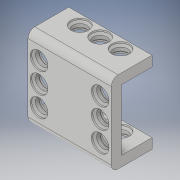
# Autodesk Inventor part: XL320_connecter
Saved by Autodesk Inventor 2018 (Build 220112000, 112)
## iProperties
Created: 2018-01-21
Part Number: XL320_connecter
Material: Generic
Document SubType Name: Modeling
Designer: wlpeng
Density: 1 g/cm^3
Appearance: Default
Author: wlpeng
Autodesk Inventor part; units mm, degrees
ref_plane "YZ Plane" through (0, 0, 0) normal (1, 0, 0) x (0, 1, 0)
ref_plane "XZ Plane" through (0, 0, 0) normal (0, 1, 0) x (-1, 0, 0)
ref_plane "XY Plane" through (0, 0, 0) normal (0, 0, 1) x (1, 0, 0)
sketch "Sketch2" plane through (0, 0, 0) normal (1, 0, 0) x (0, 1, 0)
  line L0 (3, -3) -> (3, -12)
  line L1 (3, -12) -> (0, -12)
  line L2 (0, -12) -> (0, 0)
  line L3 (21, -3) -> (3, -3)
  line L4 (0, -3) -> (0, 0)
  line L5 (21, -3) -> (21, -12)
  line L6 (21, -12) -> (24, -12)
  line L7 (24, -12) -> (24, 0)
  line L8 (24, 0) -> (0, 0)
  dimension "d2" = 24
  dimension "d3" = 3
  dimension "d4" = 12
  constraints: 18 end point, 3 parallel, 1 perpendicular
  measures "d2" distance of L2.end L7.end
  measures "d3" distance of L5.end L6.end
  measures "d4" distance of L1.end L2.end
extrude "Extrusion1" add sketch "Sketch2" along normal blind 24.5
sketch "Sketch3" plane through (0, 24, 0) normal (0, 1, 0) x (1, 0, 0)
  circle A0 centre (12.25, 9) radius 2.05
  line L0 (0, 12) -> (0, 0) projected
  line L1 (0, 0) -> (24.5, 0) projected
  line L2 (0, 12) -> (24.5, 12) projected
  dimension "d7" = 4.1
  dimension "d8" = 12.25
  dimension "d10" = 3
  constraints: 1 centre point
  measures "d7" diameter of A0
  measures "d8" distance from line of L0 A0.centre
  measures "d10" distance from line of L2 A0.centre
extrude "Extrusion2" cut sketch "Sketch3" against normal through all
sketch "Sketch4" plane through (0, 24, 0) normal (0, 1, 0) x (1, 0, 0)
  circle A0 centre (12.25, 9) radius 2.05 projected
  circle A1 centre (12.25, 9) radius 2.6
  point P0 (0, 0)
  dimension "d13" = 5.2
  constraints: 1 centre point, 1 coincident
  measures "d13" diameter of A1
extrude "Extrusion3" cut sketch "Sketch4" against normal blind 1
sketch "Sketch5" plane through (0, 21, -12) normal (0, -1, 0) x (1, 0, 0)
  circle A0 centre (12.25, 3) radius 2.6 projected
  circle A1 centre (12.25, 3) radius 2.6
  point P0 (0, 12)
  dimension "d16" = 5.2
  constraints: 1 centre point, 1 coincident
  measures "d16" diameter of A1
extrude "Extrusion4" cut sketch "Sketch5" against normal blind 1
chamfer "Chamfer1" distance 0.55 angle 45 1 edges at (9.65, 23, -9)
chamfer "Chamfer2" distance 0.55 angle 45 1 edges at (9.65, 22, -9)
sketch "Sketch6" plane through (0, 0, -12) normal (0, -1, 0) x (1, 0, 0)
  circle A0 centre (12.25, 3) radius 2.05 projected
  circle A1 centre (12.25, 3) radius 2.6
  point P0 (0, 12)
  dimension "d25" = 5.2
  constraints: 1 centre point, 1 coincident
  measures "d25" diameter of A1
extrude "Extrusion5" cut sketch "Sketch6" against normal blind 1
sketch "Sketch7" plane through (0, 3, -3) normal (0, 1, 0) x (1, 0, 0)
  circle A0 centre (12.25, 6) radius 2.6 projected
  circle A1 centre (12.25, 6) radius 2.6
  point P0 (0, -3)
  dimension "d28" = 5.2
  constraints: 1 centre point, 1 coincident
  measures "d28" diameter of A1
extrude "Extrusion6" cut sketch "Sketch7" against normal blind 1
chamfer "Chamfer3" distance 0.55 angle 45 1 edges at (9.65, 2, -9)
chamfer "Chamfer4" distance 0.55 angle 45 1 edges at (9.65, 1, -9)
pattern_linear "Rectangular Pattern1" count 2 spacing 6 along (-1, 0, 0) count 2 spacing 6 along (1, 0, 0) of "Extrusion3", "Chamfer1", "Extrusion2", "Extrusion4", "Chamfer2", "Extrusion6", "Chamfer3", "Extrusion5", "Chamfer4"
sketch "Sketch8" plane through (0, 3, -3) normal (0, 0, -1) x (-1, 0, 0)
  line L0 (0, 0) -> (0, 18) projected
  line L1 (-12.25, 9) -> (-12.25, -4.6904)
  line L2 (0, 0) -> (-24.5, 0) projected
  circle A0 centre (-3.25, 9) radius 2.05
  point P0 (0, -3)
  dimension "d44" = 12.25
  dimension "d45" = 9
  dimension "d46" = 4.1
  dimension "d47" = 9
  dimension "d49" = 18
  constraints: 2 end point, 1 centre point, 1 vertical
  measures "d44" distance from line of L0 L1.start
  measures "d45" distance from line of L2 L1.start
  measures "d46" diameter of A0
  measures "d47" distance from line of L2 A0.centre
  measures "d49" diameter of A0.centre L1
extrude "Extrusion7" cut sketch "Sketch8" against normal through all
sketch "Sketch9" plane through (0, 3, -3) normal (0, 0, -1) x (-1, 0, 0)
  circle A0 centre (-3.25, 9) radius 2.05 projected
  circle A1 centre (-3.25, 9) radius 2.6
  point P0 (0, -3)
  dimension "d52" = 5.2
  constraints: 1 centre point, 1 coincident
  measures "d52" diameter of A1
extrude "Extrusion8" cut sketch "Sketch9" against normal blind 1
sketch "Sketch10" plane through (0, 0, 0) normal (0, 0, 1) x (1, 0, 0)
  circle A0 centre (3.25, 12) radius 2.05 projected
  circle A1 centre (3.25, 12) radius 2.6
  point P0 (0, 0)
  dimension "d55" = 5.2
  constraints: 1 centre point, 1 coincident
  measures "d55" diameter of A1
extrude "Extrusion9" cut sketch "Sketch10" against normal blind 1
chamfer "Chamfer5" distance 0.55 angle 45 1 edges at (0.65, 12, -1)
chamfer "Chamfer6" distance 0.55 angle 45 1 edges at (5.85, 12, -2)
pattern_linear "Rectangular Pattern2" count 2 spacing 6 along (0, -1, 0) count 2 spacing 6 along (0, 1, 0) of "Extrusion8", "Chamfer6", "Extrusion7", "Extrusion9", "Chamfer5"
pattern_linear "Rectangular Pattern3" count 2 spacing 18 along (1, 0, 0) of "Extrusion8", "Chamfer6", "Extrusion7", "Extrusion9", "Chamfer5", "Rectangular Pattern2"
fillet "Fillet1" radius 2 1 edges at (12.25, 24, 0)
fillet "Fillet2" radius 2 1 edges at (12.25, 0, 0)
body "Solid1"
